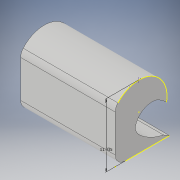
# Autodesk Inventor part: plowV2
Saved by Autodesk Inventor 2019 (Build 230136000, 136)
## iProperties
Created: 2019-04-01
Part Number: plowV2
Material: Generic
Document SubType Name: Modeling
Designer: Tesler
Density: 1 g/cm^3
Appearance: Snow
Author: Tesler
Autodesk Inventor part; units mm, degrees
ref_plane "YZ Plane" through (0, 0, 0) normal (1, 0, 0) x (0, 1, 0)
ref_plane "XZ Plane" through (0, 0, 0) normal (0, 1, 0) x (-1, 0, 0)
sketch "Sketch1" plane through (0, 0, 0) normal (1, 0, 0) x (0, 1, 0)
  line L0 (0, 0) -> (95.25, 0)
  line L1 (0, 0) -> (0, -101.6)
  line L2 (0, -101.6) -> (6.35, -90.6015)
  line L3 (0, -101.6) -> (12.7, -101.6) construction
  arc A0 (66.6929, -89.0292) -> (95.25, -12.7) centre (71.7931, -47.4307) ccw
  arc A1 (57.0991, -96.1007) -> (95.25, 0) centre (66.6458, -44.2676) ccw
  arc A2 (57.0991, -96.1007) -> (66.6929, -89.0292) centre (51.9568, -79.0806) ccw
  arc A3 (95.25, -12.7) -> (6.35, -90.6015) centre (102.2308, -110.3428) ccw
  dimension "d18" = 101.6
  dimension "d20" = 12.7
  dimension "d21" = 60
  dimension "d27" = 41.91
  dimension "d28" = 52.705
  dimension "d29" = 17.78
  dimension "d30" = 57.099
  dimension "d31" = 66.6458
  dimension "d32" = 71.7931
  dimension "d33" = 95.25
  dimension "d34" = 66.6929
  dimension "d35" = 12.7
  dimension "d36" = 96.1007
  dimension "d38" = 74.276
  constraints: 8 end point, 8 point on circle, 4 centre point, 3 horizontal, 2 vertical, 1 equal length
  measures "d18" distance of L0.start L1.end
  measures "d20" distance of L1.end L2.end
  measures "d21" angle of L3 L2
  measures "d27" radius of A0
  measures "d28" radius of A1
  measures "d29" radius of A2
  measures "d30" distance from line of L1 A1.start
  measures "d31" distance from line of L1 A1.centre
  measures "d32" distance from line of L1 A0.centre
  measures "d33" distance from line of L1 A0.end
  measures "d34" distance from line of L1 A0.start
  measures "d35" distance from line of A0.end L0
  measures "d36" distance from line of L0 A1.start
extrude "Extrusion1" add sketch "Sketch1" along normal blind 177.8
sketch "Sketch2" plane through (177.8, 0, 0) normal (1, 0, 0) x (0, 0, -1)
  arc A0 (89.0292, 66.6929) -> (12.7, 95.25) centre (47.4307, 71.7931) ccw projected
  arc A1 (12.7, 95.25) -> (90.6015, 6.35) centre (110.3428, 102.2308) ccw projected
  line L0 (0, 95.25) -> (0, 0) projected
  arc A2 (96.1007, 57.0991) -> (89.0292, 66.6929) centre (79.0806, 51.9568) ccw projected
  line L1 (0, 58.8778) -> (0, 95.25)
  line L2 (0, 0) -> (101.6, 0) projected
  arc A3 (78.465, 69.7261) -> (36.7184, 37.715) centre (69.3573, 38.3767) ccw
  arc A4 (96.1007, 57.0991) -> (78.465, 69.7261) centre (47.1123, 7.3079) ccw
  line L3 (0, 58.8778) -> (36.7184, 37.715)
  arc A5 (96.1007, 57.0991) -> (0, 95.25) centre (44.2676, 66.6458) ccw
  arc A6 (96.1007, 57.0991) -> (0, 95.25) centre (44.2676, 66.6458) ccw projected
  arc A7 (12.7, 95.25) -> (36.7184, 37.715) centre (110.3428, 102.2308) ccw
  arc A8 (89.0292, 66.6929) -> (12.7, 95.25) centre (47.4307, 71.7931) ccw
  arc A9 (96.1007, 57.0991) -> (89.0292, 66.6929) centre (79.0806, 51.9568) ccw
  dimension "d49" = 21.1628
  dimension "d50" = 32.6457
  dimension "d51" = 69.85
  dimension "d52" = 16.8716
  dimension "d53" = 59.3379
  constraints: 13 point on circle, 6 centre point, 6 concentric, 4 end point, 1 point on line, 1 vertical
  measures "d49" vertical distance of L1.start L3.end
  measures "d50" radius of A3
  measures "d51" radius of A4
  measures "d52" distance from line of A3.centre L3
  measures "d53" vertical distance of point (44.268, 66.646) A4.centre
ref_plane "Work Plane1" through (88.9, 0, 0) normal (1, 0, 0) x (0, 0, -1)
extrude "Extrusion2" add sketch "Sketch2" against normal blind 2.54
fillet "Fillet3" radius 19.05 1 edges at (176.53, 37.715, -36.7184)
mirror "Mirror1" about plane through (88.9, 0, 0) normal (1, 0, 0) of "Extrusion2", "Fillet3"
fillet "Fillet2" radius 19.05 2 edges at (88.9, 0, 0) (88.9, 95.25, 0)
sketch "Sketch3" plane through (2.54, 71.7931, -47.4307) normal (1, 0, 0) x (0, -0.3504094, -0.9365966)
  arc A0 (50.7331, 3.2921) -> (40.7482, 9.7997) centre (36.594, -7.4882) ccw projected
  arc A1 (40.7482, 9.7997) -> (-40.7482, 9.7997) centre (0, 0) ccw projected
  arc A2 (50.7331, 3.2921) -> (29.7909, 8.9388) centre (22.298, -60.5081) ccw projected
  arc A3 (50.7331, 3.2921) -> (-50.3771, 12.9226) centre (-1.1589, -5.9293) ccw projected
  arc A4 (50.7331, 3.2921) -> (40.7482, 9.7997) centre (36.594, -7.4882) ccw
  arc A5 (41.3731, 6.6868) -> (40.7482, 9.7997) centre (0, 0) ccw
  arc A6 (50.7331, 3.2921) -> (29.7909, 8.9388) centre (22.298, -60.5081) ccw projected
  arc A7 (-35.8187, -21.7593) -> (-43.5602, -37.2333) centre (22.298, -60.5081) ccw
  arc A8 (50.7331, 3.2921) -> (41.3731, 6.6868) centre (22.298, -60.5081) ccw
  point P0 (-19.2665, -83.8613)
  constraints: 14 point on circle, 4 centre point, 3 concentric
extrude "Extrusion3" add sketch "Sketch3" along normal up to next
sketch "Sketch4" plane through (177.8, 0, 0) normal (1, 0, 0) x (0, 0, -1)
  arc A0 (96.1007, 57.0991) -> (4.7759, 101.5489) centre (44.2676, 66.6458) ccw projected
  line L0 (19.05, 0) -> (101.6, 0) projected
  arc A1 (96.1007, 57.0991) -> (4.7759, 101.5489) centre (44.2676, 66.6458) ccw projected
  point P0 (0, 0)
  point P1 (44.2676, 119.3508)
  dimension "d57" = 119.3508
  constraints: 1 point on circle
  measures "d57" distance from line of L0 point (44.268, 119.351)
body "Solid1"
